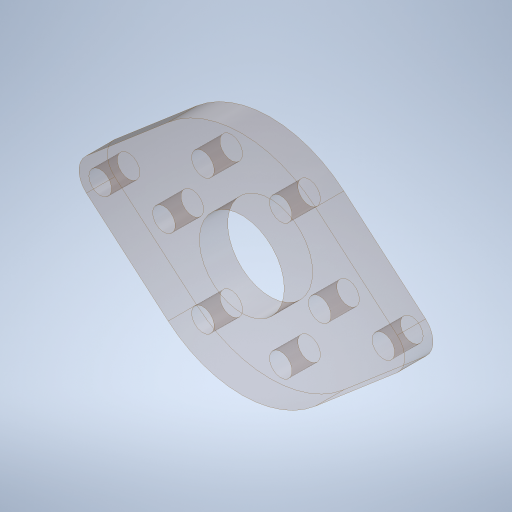
# Autodesk Inventor part: GP8-003
Saved by Autodesk Inventor 2023.4 (Build 274418000, 418)
## iProperties
Created: 2025-02-24
Part Number: GP8-003
Material: Polycarbonate, Smoke
Document SubType Name: Modeling
Designer: dlangdon
Density: 1.2 g/cm^3
Appearance: Polycarbonate - Smoked
Author: dlangdon
Autodesk Inventor part; units mm, degrees
ref_plane "YZ Plane" through (0, 0, 0) normal (1, 0, 0) x (0, 1, 0)
ref_plane "XZ Plane" through (0, 0, 0) normal (0, 1, 0) x (-1, 0, 0)
ref_plane "XY Plane" through (0, 0, 0) normal (0, 0, 1) x (1, 0, 0)
sketch "Sketch1" plane through (0, 0, 0) normal (0, 0, 1) x (1, 0, 0)
  circle A0 centre (0, 0) radius 9.525
  circle A1 centre (0, 0) radius 25.4 construction
  circle A2 centre (-31.75, 0) radius 4.7625 construction
  circle A3 centre (31.75, 0) radius 4.7625 construction
  circle A4 centre (0, 0) radius 17.4625 construction
  line L0 (-16.51, 19.3023) -> (-34.8456, 3.6192)
  line L1 (-34.8456, -3.6192) -> (-16.51, -19.3023)
  line L2 (16.51, -19.3023) -> (34.8456, -3.6192)
  line L3 (34.8456, 3.6192) -> (16.51, 19.3023)
  arc A5 (-34.8456, 3.6192) -> (-34.8456, -3.6192) centre (-31.75, 0) ccw
  arc A6 (-16.51, -19.3023) -> (16.51, -19.3023) centre (0, 0) ccw
  arc A7 (34.8456, -3.6192) -> (34.8456, 3.6192) centre (31.75, 0) ccw
  arc A8 (16.51, 19.3023) -> (-16.51, 19.3023) centre (0, 0) ccw
  line L4 (-31.75, 0) -> (31.75, 0) construction
  point P0 (-17.4625, 0)
  point P1 (-8.7313, -15.123)
  point P2 (8.7312, -15.123)
  point P3 (17.4625, 0)
  point P4 (8.7313, 15.123)
  point P5 (-8.7312, 15.123)
  point P6 (-33.4211, -3.4732)
  dimension "d3" = 34.925
  dimension "d0" = 19.05
  dimension "d1" = 50.8
  dimension "d2" = 9.525
  dimension "d6" = 360
  dimension "d17" = 63.5
  constraints: 16 point on circle, 10 coincident, 10 end point, 8 centre point, 8 tangent, 4 horizontal alignment, 2 equal radius, 1 horizontal, 1 midpoint, 9 other
  measures "d0" diameter of A0
  measures "d1" diameter of A1
  measures "d2" diameter of A2
  measures "d17" distance of L4.start L4.end
extrude "Extrusion1" add sketch "Sketch1" along normal blind 6.35
hole "Hole1" at (-17.4625, 0, 0) at (-8.7313, -15.123, 0) at (8.7312, -15.123, 0) at (17.4625, 0, 0) at (8.7313, 15.123, 0) at (-8.7312, 15.123, 0) at (-31.75, 0, 0) at (31.75, 0, 0) direction (0, 0, 1) diameter 5.1054 end through all clearance for "Flat Head Machine Screw (82)" size "#10" standard "Ansi Unified Screw Threads"
body "Solid1"
